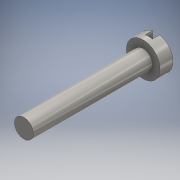
# Autodesk Inventor part: screw27x4mm
Saved by Autodesk Inventor 2016 (Build 200138000, 138)
## iProperties
Created: 2016-06-04
Part Number: screw27x4mm
Material: Stainless Steel
Document SubType Name: Modeling
Designer: hesaon
Density: 8 g/cm^3
Appearance: Semi-Polished
Author: hesaon
Autodesk Inventor part; units mm, degrees
ref_plane "YZ Plane" through (0, 0, 0) normal (1, 0, 0) x (0, 1, 0)
ref_plane "XZ Plane" through (0, 0, 0) normal (0, 1, 0) x (-1, 0, 0)
ref_plane "XY Plane" through (0, 0, 0) normal (0, 0, 1) x (1, 0, 0)
sketch "Sketch1" plane through (0, 0, 0) normal (0, 1, 0) x (-1, 0, 0)
  circle A0 centre (0, 0) radius 1.95
  dimension "d0" = 3.9
  constraints: 1 centre point, 1 coincident
  measures "d0" diameter of A0
extrude "Extrusion1" add sketch "Sketch1" along normal blind 24.8
sketch "Sketch2" plane through (0, 24.8, 0) normal (0, 1, 0) x (1, 0, 0)
  circle A0 centre (0, 0) radius 3.5
  dimension "d3" = 7
  constraints: 1 centre point, 1 coincident
  measures "d3" diameter of A0
extrude "Extrusion2" add sketch "Sketch2" along normal blind 2.7
sketch "Sketch3" plane through (0, 27.5, 0) normal (0, 1, 0) x (1, 0, 0)
  line L0 (0.75, -8) -> (-0.75, -8)
  line L1 (-0.75, -8) -> (-0.75, 8)
  line L2 (-0.75, 8) -> (0.75, 8)
  line L3 (0.75, 8) -> (0.75, -8)
  line L4 (0.75, -8) -> (-0.75, 8) construction
  line L5 (-0.75, -8) -> (0.75, 8) construction
  point P0 (0, 0)
  dimension "d6" = 1.5
  dimension "d7" = 16
  constraints: 12 end point, 2 midpoint, 2 parallel, 1 horizontal, 1 perpendicular
  measures "d6" distance of L1.end L2.end
  measures "d7" distance of L0.end L1.end
extrude "Extrusion3" cut sketch "Sketch3" against normal blind 1.5
body "Solid1"
